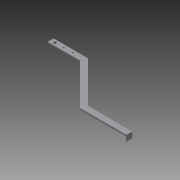
# Autodesk Inventor part: Z-PickupArm-R
Saved by Autodesk Inventor 2013 (Build 170138000, 138)
## iProperties
Created: 2014-01-22
Part Number: Z-PickupArm-R
Material: Generic
Document SubType Name: Modeling
Designer: Jarod
Density: 1 g/cm^3
Author: Jarod
Autodesk Inventor part; units mm, degrees
ref_plane "YZ Plane" through (0, 0, 0) normal (1, 0, 0) x (0, 1, 0)
ref_plane "XZ Plane" through (0, 0, 0) normal (0, 1, 0) x (-1, 0, 0)
ref_plane "XY Plane" through (0, 0, 0) normal (0, 0, 1) x (1, 0, 0)
sketch "Sketch1" plane through (0, 0, 0) normal (0, 1, 0) x (-1, 0, 0)
  line L0 (0, 0) -> (-133.35, 0)
  line L1 (-133.35, 0) -> (-133.35, 25.4)
  line L2 (-133.35, 25.4) -> (0, 25.4)
  line L3 (0, 25.4) -> (0, 0)
  line L4 (-133.35, 25.4) -> (-143.871, 0)
  line L5 (-133.35, 25.4) -> (-105.8572, 25.4) construction
  line L6 (-133.35, 25.4) -> (-151.3105, 7.4395)
  line L7 (-133.35, 25.4) -> (-107.95, 25.4) construction
  line L8 (-151.3105, 7.4395) -> (-143.871, 0)
  line L9 (-133.35, 25.4) -> (-151.3105, 7.4395)
  line L10 (-151.3105, 7.4395) -> (-323.48, 179.609)
  line L11 (-323.48, 179.609) -> (-305.5195, 197.5695)
  line L12 (-305.5195, 197.5695) -> (-133.35, 25.4)
  circle A0 centre (-12.7, 12.7) radius 6.35
  line L13 (-323.48, 179.609) -> (-513.98, 179.609)
  line L14 (-513.98, 179.609) -> (-513.98, 205.009)
  line L15 (-513.98, 205.009) -> (-323.48, 205.009)
  line L16 (-323.48, 205.009) -> (-323.48, 179.609)
  line L17 (-323.48, 179.609) -> (-312.959, 205.009)
  line L18 (-312.959, 205.009) -> (-323.48, 205.009)
  line L19 (-312.959, 205.009) -> (-305.5195, 197.5695)
  line L20 (-133.35, 0) -> (-143.871, 0)
  dimension "d0" = 133.35
  dimension "d1" = 25.4
  dimension "d2" = 112.5
  dimension "d3" = 25.4
  dimension "d4" = 135
  dimension "d5" = 243.4844
  dimension "d6" = 12.7
  dimension "d7" = 190.5
  dimension "d8" = 25.4
  constraints: 42 end point, 7 parallel, 6 perpendicular, 4 horizontal, 2 equal length, 1 centre point
  measures "d0" distance of L1.end L2.end
  measures "d1" distance of L0.end L1.end
  measures "d2" angle of L4 L5
  measures "d3" distance of L1.end L6.end
  measures "d4" angle of L6 L7
  measures "d5" distance of L6.end L10.end
  measures "d6" diameter of A0
  measures "d7" distance of L14.end L15.end
  measures "d8" distance of L13.end L14.end
extrude "Extrusion1" add sketch "Sketch1" along normal blind 6.35
sketch "Sketch2" plane through (513.98, 0, 205.009) normal (1, 0, 0) x (0, 0, -1)
  line L0 (0, 6.35) -> (25.4, 6.35)
  line L1 (25.4, 6.35) -> (25.4, -19.05)
  line L2 (25.4, -19.05) -> (0, -19.05)
  line L3 (0, -19.05) -> (0, 6.35)
  point P0 (205.009, 0)
  dimension "d11" = 25.4
  dimension "d12" = 25.4
  constraints: 8 end point, 2 parallel, 1 horizontal, 1 perpendicular
  measures "d11" distance of L1.end L2.end
  measures "d12" distance of L0.end L1.end
extrude "Extrusion2" add sketch "Sketch2" along normal blind 1.5875
sketch "Sketch3" plane through (0, 0, 0) normal (-1, 0, 0) x (0, 0, 1)
  line L0 (0, 0) -> (25.4, 0) projected
  line L1 (25.4, 0) -> (25.4, 6.35) projected
  line L2 (0, 6.35) -> (25.4, 6.35) projected
  line L3 (0, 0) -> (0, 6.35) projected
extrude "Extrusion3" add sketch "Sketch3" along normal blind 44.45
sketch "Sketch6" plane through (0, 6.35, 0) normal (0, 1, 0) x (1, 0, 0)
  circle A0 centre (12.7, -12.7) radius 6.35 projected
  line L0 (323.48, -179.609) -> (515.5675, -179.609) projected
  line L1 (12.7, -12.7) -> (12.7, -6.35)
  line L2 (16.3662, -6.35) -> (20.0323, -12.7)
  line L3 (20.0323, -12.7) -> (16.3662, -19.05)
  line L4 (16.3662, -19.05) -> (9.0338, -19.05)
  line L5 (9.0338, -19.05) -> (5.3677, -12.7)
  line L6 (5.3677, -12.7) -> (9.0338, -6.35)
  line L7 (9.0338, -6.35) -> (16.3662, -6.35)
  point P0 (0, 0)
  constraints: 14 end point, 1 coincident, 1 midpoint, 1 perpendicular, 1 vertical alignment, 14 other
extrude "Extrusion5" cut sketch "Sketch6" against normal blind 6.35 contours A0 L2 L3 | A0 L7 L2 | L3 L4 A0 | A0 L6 L7 | L4 L5 A0 | A0 L5 L6
sketch "Sketch8" plane through (0, 6.35, 0) normal (0, 1, 0) x (1, 0, 0)
  line L0 (143.871, 0) -> (-44.45, 0) projected
  line L1 (-44.45, -25.4) -> (-44.45, 0) projected
  line L2 (323.48, -179.609) -> (515.5675, -179.609) projected
  line L3 (-44.45, -12.7) -> (12.7, -12.7)
  line L4 (12.7, -12.7) -> (12.7, 0)
  line L5 (12.7, -12.7) -> (-25.4, -12.7)
  line L6 (-25.4, -12.7) -> (50.8, -12.7)
  circle A0 centre (-25.4, -12.7) radius 3.175
  circle A1 centre (50.8, -12.7) radius 3.175
  point P0 (0, 0)
  dimension "d29" = 57.15
  dimension "d30" = 38.1
  dimension "d31" = 76.2
  dimension "d32" = 0
  dimension "d33" = 6.35
  dimension "d34" = 6.35
  constraints: 8 end point, 2 centre point, 2 coincident, 2 point on line, 1 collinear, 1 midpoint, 1 parallel, 1 perpendicular
  measures "d29" distance of L3.start L3.end
  measures "d30" distance of L3.end L5.end
  measures "d31" distance of L5.end L6.end
  measures "d32" distance between parallel lines of L6 L5
  measures "d33" diameter of A0
  measures "d34" diameter of A1
extrude "Extrusion7" cut sketch "Sketch8" against normal blind 25.4 contours A0 L3 | L3 A0 | A1
sketch "Sketch9" plane through (0, 6.35, 0) normal (0, 1, 0) x (1, 0, 0)
  circle A0 centre (50.8, -12.7) radius 3.175 projected
  circle A1 centre (-25.4, -12.7) radius 3.175 projected
  line L0 (-44.45, 0) -> (0, 0)
  line L1 (0, 0) -> (0, -25.4)
  line L2 (0, -25.4) -> (-44.45, -25.4)
  line L3 (-44.45, -25.4) -> (-44.45, 0)
  line L4 (0, -12.7) -> (12.7, -12.7)
  line L5 (12.7, -12.7) -> (50.8, -12.7)
  line L6 (50.8, -12.7) -> (88.9, -12.7)
  line L7 (50.8, -12.7) -> (88.9, -12.7) construction
  circle A2 centre (88.9, -12.7) radius 3.175
  dimension "d37" = 44.45
  dimension "d38" = 25.4
  dimension "d39" = 38.1
  dimension "d40" = 0
  dimension "d41" = 6.35
  constraints: 16 end point, 3 equal length, 2 horizontal, 2 perpendicular, 1 centre point, 1 coincident, 1 collinear, 1 midpoint
  measures "d37" distance of L1.end L2.end
  measures "d38" distance of L0.end L1.end
  measures "d39" distance of L5.end L6.end
  measures "d40" distance between parallel lines of L6 L7
  measures "d41" diameter of A2
extrude "Extrusion8" cut sketch "Sketch9" against normal blind 25.4 contours L0 L1 L2 L3 | A2
sketch "Sketch10" plane through (0, 6.35, 0) normal (-1, 0, 0) x (0, 0, 1)
  line L0 (25.4, -6.35) -> (0, -6.35) projected
  line L1 (25.4, 0) -> (25.4, -6.35) projected
  line L2 (0, 0) -> (25.4, 0) projected
  line L3 (0, -6.35) -> (0, 0) projected
extrude "Extrusion9" add sketch "Sketch10" along normal blind 6.35
sketch "Sketch11" plane through (0, 6.35, 0) normal (0, 1, 0) x (1, 0, 0)
  line L0 (-6.35, -25.4) -> (-6.35, 0) projected
  line L1 (5.3677, -12.7) -> (9.0338, -6.35) projected
  line L2 (9.0338, -6.35) -> (16.3662, -6.35) projected
  line L3 (16.3662, -6.35) -> (20.0323, -12.7) projected
  line L4 (20.0323, -12.7) -> (16.3662, -19.05) projected
  line L5 (16.3662, -19.05) -> (9.0338, -19.05) projected
  line L6 (9.0338, -19.05) -> (5.3677, -12.7) projected
  line L7 (-6.35, -12.7) -> (12.7, -12.7)
  line L8 (12.7, -12.7) -> (6.35, -12.7)
  line L9 (12.7, -12.7) -> (19.05, -12.7) construction
  line L10 (6.35, -12.7) -> (9.525, -7.2007)
  line L11 (9.525, -7.2007) -> (15.875, -7.2007)
  line L12 (15.875, -7.2007) -> (19.05, -12.7)
  line L13 (19.05, -12.7) -> (15.875, -18.1993)
  line L14 (15.875, -18.1993) -> (9.525, -18.1993)
  line L15 (9.525, -18.1993) -> (6.35, -12.7)
  point P0 (0, 0)
  dimension "d46" = 6.35
  dimension "d47" = 180
  constraints: 18 end point, 2 collinear, 1 coincident, 1 horizontal, 1 midpoint, 1 parallel, 13 other
  measures "d46" distance of L7.end L8.end
  measures "d47" angle of L8 L9
extrude "Extrusion10" add sketch "Sketch11" against normal blind 6.35
body "Solid1"
